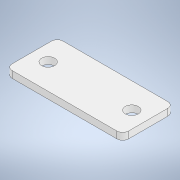
# Autodesk Inventor part: SP11V1 Planchuela Baranda
Saved by Autodesk Inventor 2021.2 (Build 252289000, 289)
## iProperties
Created: 2026-06-02
Part Number: SP11V1 Planchuela Baranda
Material: Acero, carbono
Document SubType Name: Modeling
Designer: nelso
Density: 7.85 g/cm^3
Appearance: Blanco
Author: nelso
Autodesk Inventor part; units mm, degrees
ref_plane "YZ Plane" through (0, 0, 0) normal (1, 0, 0) x (0, 1, 0)
ref_plane "XZ Plane" through (0, 0, 0) normal (0, 1, 0) x (-1, 0, 0)
ref_plane "XY Plane" through (0, 0, 0) normal (0, 0, 1) x (1, 0, 0)
sketch "Sketch1" plane through (0, 0, 0) normal (0, 1, 0) x (-1, 0, 0)
  line L0 (-40, 17.5) -> (40, 17.5)
  line L1 (40, 17.5) -> (40, -17.5)
  line L2 (40, -17.5) -> (-40, -17.5)
  line L3 (-40, -17.5) -> (-40, 17.5)
  line L4 (-40, 17.5) -> (40, -17.5) construction
  line L5 (40, 17.5) -> (-40, -17.5) construction
  point P0 (0, 0)
  point P1 (0, 0)
  dimension "d10" = 80
  dimension "d11" = 35
  constraints: 12 end point, 2 parallel, 1 coincident, 1 horizontal, 1 midpoint, 1 perpendicular
  measures "d10" distance of L1.end L2.end
  measures "d11" distance of L0.end L1.end
extrude "Extrusion3" add sketch "Sketch1" along normal mid plane 4.7
sketch "Sketch3" plane through (0, 2.35, 0) normal (0, 1, 0) x (1, 0, 0)
  line L0 (-40, 17.5) -> (-40, -17.5) projected
  circle A0 centre (-28.75, 0) radius 4.5
  circle A1 centre (0, 0) radius 17.5
  line L1 (40, -17.5) -> (40, 17.5) projected
  circle A2 centre (28.75, 0) radius 4.5
  line L2 (17.5, 0) -> (17.5, -17.5)
  line L3 (-40, -17.5) -> (40, -17.5) projected
  dimension "d18" = 35
  dimension "d15" = 9
  dimension "d17" = 9
  dimension "d19" = 22.5
  dimension "d20" = 11.25
  dimension "d21" = 11.25
  constraints: 2 centre point, 2 end point, 2 vertical, 1 coincident, 1 horizontal alignment, 1 point on line, 2 other
  measures "d15" diameter of A0
  measures "d17" diameter of A2
  measures "d19" distance between parallel lines of L1 L2
  measures "d20" distance from line of L1 A2.centre
  measures "d21" distance from line of A0.centre L0
extrude "Extrusion4" cut sketch "Sketch3" against normal through all contours A0 | A2
fillet "Fillet1" radius 4 4 edges at (-40, 0, 17.5) (40, 0, 17.5) (40, 0, -17.5) (-40, 0, -17.5)
equation "\"d15\" = d17"
equation "\"d20\" = 0.5 * d19"
equation "\"d21\" = d20"
body "Solid2"
